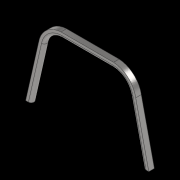
# Autodesk Inventor part: McCrea_noha_walle
Saved by Autodesk Inventor 2021 (Build 250183000, 183)
## iProperties
Created: 2022-01-17
Part Number: McCrea_noha_walle
Material: Generic
Document SubType Name: Modeling
Designer: student
Density: 1 g/cm^3
Appearance: Default
Author: student
Autodesk Inventor part; units mm, degrees
ref_plane "YZ Plane" through (0, 0, 0) normal (1, 0, 0) x (0, 1, 0)
ref_plane "XZ Plane" through (0, 0, 0) normal (0, 1, 0) x (-1, 0, 0)
ref_plane "XY Plane" through (0, 0, 0) normal (0, 0, 1) x (1, 0, 0)
sketch "Sketch1" plane through (0, 0, 0) normal (0, 0, 1) x (1, 0, 0)
  line L0 (0, 41) -> (0, -27)
  line L1 (-30.5054, 0) -> (-23.3898, 31.222)
  line L2 (-13.6398, 39) -> (0, 39)
  arc A0 (-13.6398, 39) -> (-23.3898, 31.222) centre (-13.6398, 29) ccw
  line L3 (0, -40.6) -> (0, 54.6) projected
  line L4 (-36.6064, 0) -> (6.1011, 0) projected
  point P0 (0, 0)
  point P1 (-21.6172, 39)
  dimension "d2" = 21.6172
  dimension "d3" = 40
  dimension "d4" = 10
  dimension "d6" = 39
  constraints: 6 end point, 3 point on line, 2 point on circle, 2 tangent, 1 centre point, 1 collinear, 1 horizontal alignment, 1 perpendicular, 1 vertical
  measures "d2" distance of point (-21.617, 39) L2.end
  measures "d3" distance of L1.start point (-21.617, 39)
  measures "d4" radius of A0
  measures "d6" distance between parallel lines of L2 L4
sketch "Sketch2" plane through (0, 0, 0) normal (0, 1, 0) x (-1, 0, 0)
  circle A0 centre (32.0053, 0) radius 1.5
  line L0 (33.5053, 1.5) -> (32.0053, 1.5)
  line L1 (32.0053, -1.5) -> (33.5053, -1.5)
  line L2 (33.5053, -1.5) -> (33.5053, 1.5)
  line L3 (40.2063, 0) -> (-6.7011, 0) projected
  point P0 (0, 0)
  point P1 (33.5053, 0)
  dimension "d5" = 3
  constraints: 6 end point, 2 point on circle, 2 tangent, 1 centre point, 1 horizontal, 1 parallel, 1 perpendicular
  measures "d5" diameter of A0
sweep "Sweep1" add profiles "Sketch2" path "Sketch1" path curves L1 A0 L2
mirror "Mirror1" about plane through (0, 0, 0) normal (1, 0, 0) of "Sweep1"
sketch "Sketch4" plane through (0, 0, 0) normal (1, 0, 0) x (0, 1, 0)
  line L0 (39, 0.0174) -> (39, -0.0174) projected
  ellipse E0 centre (40.4624, 0) end of major axis (40.4624, 1.5) minor radius 1.4625 (40.4624, 1.5) -> (39, 0.0174) ccw projected
  line L1 (40.4624, 1.5) -> (41.9249, 1.5)
  line L2 (41.9249, 1.5) -> (41.9249, -1.5)
  line L3 (41.9249, -1.5) -> (40.4624, -1.5)
  line L4 (31.222, 1.5) -> (31.222, -1.5) projected
  ellipse E1 centre (40.4624, 0) end of major axis (40.4624, 1.5) minor radius 1.4625 (40.4624, 1.5) -> (40.4624, -1.5) ccw projected
  line L5 (31.222, -1.5) -> (40.4624, -1.5) projected
  line L6 (31.222, 1.5) -> (40.4624, 1.5) projected
  line L7 (41.9249, 1.5) -> (40.4624, 1.5) projected
  line L8 (41.9249, -1.5) -> (41.9249, 1.5) projected
  line L9 (40.4624, -1.5) -> (41.9249, -1.5) projected
  ellipse E2 centre (40.4624, 0) end of major axis (40.4624, 1.5) minor radius 1.4625 (39, -0.0174) -> (40.4624, -1.5) ccw projected
  point P0 (0, 0)
  point P1 (41.9249, 0)
  constraints: 6 end point, 3 horizontal, 2 perpendicular, 1 vertical, 5 other
extrude "Extrusion1" add sketch "Sketch4" along normal mid plane 27 contours E0 L1 L2 L3 E1 L0
body "Solid1"
